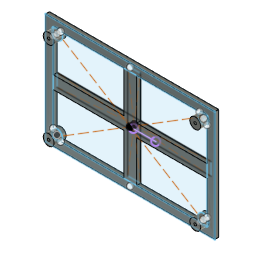
body 3 (Autodesk Fusion 360 design; units mm, degrees)
Autodesk Fusion 360 part; units mm, degrees
sketch "Sketch1" plane through (0, 0, 0) normal (0, 1, 0) x (1, 0, 0)
  line L0 (60.3, -37.35) -> (-60.3, -37.35)
  line L1 (-60.3, -37.35) -> (-60.3, 31.2432)
  line L2 (-60.3, 37.35) -> (60.3, 37.35)
  line L3 (60.3, 37.35) -> (60.3, -37.35)
  line L4 (60.3, -37.35) -> (-60.3, 37.35) construction
  line L5 (-60.3, -37.35) -> (60.3, 37.35) construction
  line L6 (-66.3, 43.35) -> (66.3, 43.35)
  line L7 (66.3, 43.35) -> (66.3, -43.35)
  line L8 (66.3, -43.35) -> (-66.3, -43.35)
  line L9 (-66.3, -43.35) -> (-66.3, 43.35)
  line L10 (-60.3, -37.35) -> (-54.5, -37.35)
  line L11 (-60.3, -31.35) -> (-60.3, -37.35)
  line L12 (60.3, -37.35) -> (54.5, -37.35)
  line L13 (60.3, -31.35) -> (60.3, -37.35)
  line L14 (-60.3, 37.35) -> (-54.5, 37.35)
  line L15 (-60.3, 31.35) -> (-60.3, 37.35)
  line L16 (60.3, 37.35) -> (54.5, 37.35)
  line L17 (60.3, 31.35) -> (60.3, 37.35)
  circle A0 centre (-57.4, -34.35) radius 1
  circle A1 centre (57.4, -34.35) radius 1
  line L18 (2.5, 0) -> (20, 0)
  circle A2 centre (57.4, 34.35) radius 1
  circle A3 centre (-57.4, 34.35) radius 1
  circle A4 centre (0, -40.35) radius 1
  circle A5 centre (0, 40.35) radius 1
  circle A6 centre (57.4, -34.35) radius 4.25
  circle A7 centre (57.4, 34.35) radius 4.25
  circle A8 centre (-57.4, 34.35) radius 4.25
  circle A9 centre (-57.4, -34.35) radius 4.25
  point P0 (-57.4, 34.35)
  dimension "d1" = 120.6
  dimension "d2" = 74.7
  dimension "d6" = 5.8
  dimension "d7" = 6
  dimension "d8" = 5.8
  dimension "d9" = 6
  dimension "d10" = 5.8
  dimension "d11" = 6
  dimension "d12" = 5.8
  dimension "d13" = 6
  dimension "d16" = 2
  dimension "d17" = 2
  dimension "d18" = 2
  dimension "d22" = 2
  dimension "d23" = 8.5
  dimension "d24" = 8.5
  dimension "d25" = 8.5
  dimension "d26" = 8.5
  constraint horizontal L0
  constraint perpendicular L0 L1
  constraint parallel L0 L2
  constraint parallel L1 L3
  constraint coincident L4 origin
  constraint coincident L5 origin
  constraint horizontal L10
  constraint vertical L11
  constraint horizontal L12
  constraint vertical L13
  constraint horizontal L14
  constraint vertical L15
  constraint horizontal L16
  constraint vertical L17
  constraint symmetric A0.centre L18 P0
  constraint symmetric A1 L18 A2
  constraint coincident P0 A3.centre
  constraint symmetric L18 A4 A5
  constraint concentric A1 A6
  constraint concentric A2 A7
  constraint concentric A0 A9
  constraint coincident A8 L1.end
  measures "d1" distance of L2.start L2.end
  measures "d2" distance of L0.end L2.start
  measures "d6" distance of L0.end L10.end
  measures "d7" distance of L0.end L11.start
  measures "d8" distance of L0.start L12.end
  measures "d9" distance of L0.start L13.start
  measures "d10" distance of L2.start L14.end
  measures "d11" distance of L2.start L15.start
  measures "d12" distance of L2.end L16.end
  measures "d13" distance of L2.end L17.start
  measures "d16" diameter of A0
  measures "d17" diameter of A1
  measures "d18" diameter of A3
  measures "d22" diameter of A4
  measures "d23" diameter of A6
  measures "d24" diameter of A7
  measures "d25" diameter of A8
  measures "d26" diameter of A9
extrude "Extrude1" add sketch "Sketch1" along normal blind 3 contours L0 L3 L12 L13 A6 | L0 L3 L12 L13 A6 | L0 L1 L2 L3 A6 A7 A8 A9 | L0 L1 L10 L11 A9 | L0 L1 L10 L11 A9 | L2 L3 L16 L17 A7 | L2 L3 L16 L17 A7 | A8 | L6 L7 L8 L9 | A0 | A1 | A2 | A3 | A4 | A5
extrude "Extrude3" cut sketch "Sketch1" along normal blind 10 contours A0 | A1 | A2 | A3
extrude "Extrude4" add sketch "Sketch1" against normal blind 6.5 contours L0 L3 L12 L13 A6 | L0 L3 L12 L13 A6 | L0 L1 L10 L11 A9 | L0 L1 L10 L11 A9 | L2 L3 L16 L17 A7 | L2 L3 L16 L17 A7 | A8
sketch "Sketch2" plane through (0, 0, 0) normal (0, 1, 0) x (1, 0, 0)
extrude "Extrude5" cut sketch "Sketch1" along normal blind 10 contours L0 L1 L2 L3 A6 A7 A8 A9
sketch "Sketch3" plane through (0, 3, 0) normal (0, 1, 0) x (-1, 0, 0)
  arc A0 (54.3896, 37.35) -> (60.3, 31.2432) centre (57.4, 34.35) ccw
  line L0 (60.3, 31.2432) -> (60.3, -31.2432)
  arc A1 (60.3, -31.2432) -> (54.3896, -37.35) centre (57.4, -34.35) ccw
  line L1 (54.3896, -37.35) -> (-54.3896, -37.35)
  arc A2 (-54.3896, -37.35) -> (-60.3, -31.2432) centre (-57.4, -34.35) ccw
  line L2 (-60.3, -31.2432) -> (-60.3, 31.2432)
  arc A3 (-60.3, 31.2432) -> (-54.3896, 37.35) centre (-57.4, 34.35) ccw
  line L3 (-54.3896, 37.35) -> (54.3896, 37.35)
  circle A4 centre (57.4, -34.35) radius 1
  circle A5 centre (57.4, 34.35) radius 1
  circle A6 centre (-57.4, -34.35) radius 1
  circle A7 centre (-57.4, 34.35) radius 1
  line L4 (66.3, 43.35) -> (-66.3, 43.35)
  line L5 (-66.3, 43.35) -> (-66.3, -43.35)
  line L6 (-66.3, -43.35) -> (66.3, -43.35)
  line L7 (66.3, -43.35) -> (66.3, 43.35)
  line L8 (-5, -37.35) -> (5, -37.35)
  line L9 (5, -37.35) -> (5, 37.35)
  line L10 (5, 37.35) -> (-5, 37.35)
  line L11 (-5, 37.35) -> (-5, -37.35)
  line L12 (-5, -37.35) -> (5, 37.35) construction
  line L13 (5, -37.35) -> (-5, 37.35) construction
  line L14 (60.3, 5) -> (-60.3, 5)
  line L15 (-60.3, 5) -> (-60.3, -5)
  line L16 (-60.3, -5) -> (60.3, -5)
  line L17 (60.3, -5) -> (60.3, 5)
  line L18 (60.3, 5) -> (-60.3, -5) construction
  line L19 (-60.3, 5) -> (60.3, -5) construction
  dimension "d31" = 10
  dimension "d32" = 10
  constraint horizontal L8
  constraint perpendicular L8 L9
  constraint parallel L8 L10
  constraint parallel L9 L11
  constraint coincident L12 origin
  constraint coincident L13 origin
  constraint horizontal L14
  constraint perpendicular L14 L15
  constraint parallel L14 L16
  constraint parallel L15 L17
  constraint coincident L18 origin
  constraint coincident L19 origin
  measures "d31" distance of L9.end L10.end
  measures "d32" distance of L14.end L15.end
extrude "Extrude6" add sketch "Sketch3" against normal blind 3 contours L3 L9 L10 L11 L14 | L0 L9 L14 L16 L17 | L9 L11 L14 L16 | L2 L11 L14 L15 L16 | L1 L8 L9 L11 L16
